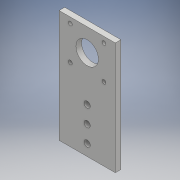
# Autodesk Inventor part: MotorPlate
Saved by Autodesk Inventor 2017 (Build 210142000, 142)
## iProperties
Created: 2017-03-12
Part Number: MotorPlate
Material: Generic
Document SubType Name: Modeling
Designer: umr
Density: 1 g/cm^3
Appearance: Default
Author: umr
Autodesk Inventor part; units mm, degrees
ref_plane "YZ Plane" through (0, 0, 0) normal (1, 0, 0) x (0, 1, 0)
ref_plane "XZ Plane" through (0, 0, 0) normal (0, 1, 0) x (-1, 0, 0)
ref_plane "XY Plane" through (0, 0, 0) normal (0, 0, 1) x (1, 0, 0)
sketch "Sketch1" plane through (0, 0, 0) normal (0, 1, 0) x (-1, 0, 0)
  line L0 (0, 0) -> (50, 0)
  line L1 (50, 0) -> (50, -100)
  line L2 (50, -100) -> (0, -100)
  line L3 (0, -100) -> (0, 0)
  dimension "d0" = 50
  dimension "d1" = 100
  constraints: 8 end point, 2 parallel, 1 horizontal, 1 perpendicular
  measures "d0" distance of L1.end L2.end
  measures "d1" distance of L0.end L1.end
extrude "Extrusion1" add sketch "Sketch1" along normal blind 5
sketch "Sketch2" plane through (0, 5, 0) normal (0, 1, 0) x (1, 0, 0)
  line L0 (-50, 0) -> (0, 0) projected
  line L1 (0, 0) -> (0, 100) projected
  line L2 (0, 100) -> (-50, 100) projected
  line L3 (-50, 100) -> (-50, 0) projected
  circle A0 centre (-25, 90) radius 2.75
  circle A1 centre (-25, 75) radius 2.75
  circle A2 centre (-25, 60) radius 2.75
  circle A3 centre (-40, 5) radius 1.75
  circle A4 centre (-40, 35) radius 1.75
  circle A5 centre (-10, 5) radius 1.75
  circle A6 centre (-10, 35) radius 1.75
  circle A7 centre (-25, 20) radius 10
  dimension "d4" = 5.5
  dimension "d5" = 100
  dimension "d6" = 10
  dimension "d7" = 25
  dimension "d10" = 15
  dimension "d16" = 3.5
  dimension "d19" = 30
  dimension "d22" = 30
  dimension "d25" = 5
  dimension "d26" = 10
  dimension "d33" = 20
  dimension "d34" = 15
  dimension "d35" = 15
  constraints: 8 centre point, 2 vertical, 1 horizontal, 10 other
  measures "d4" diameter of A0
  measures "d5" distance of L2.end L0.start
  measures "d6" distance from line of L2 A0.centre
  measures "d7" distance from line of L3 A0.centre
  measures "d10" distance of A0.centre A1.centre
  measures "d16" diameter of A3
  measures "d19" distance of A3.centre A4.centre
  measures "d22" distance of A3.centre A5.centre
  measures "d25" distance from line of L0 A3.centre
  measures "d26" distance from line of L1 A5.centre
  measures "d33" diameter of A7
  measures "d34" horizontal distance of A5.centre A7.centre
  measures "d35" horizontal distance of A6.centre A7.centre
extrude "Extrusion3" cut sketch "Sketch2" against normal blind 5 contours A0 | A1 | A2 | A3 | A4 | A5 | A6 | A7
equation "\"d7\" = 0.5 * d29"
equation "\"d22\" = d19"
equation "\"d34\" = 0.5 * d19"
equation "\"d35\" = d34"
equation "\"d29\" = 50"
body "Solid1"
